Autodesk Fusion 360 part; units mm, degrees
note: some values were not read from the file. Set by a fixed rule: which face or edge a step refers to.
(part 2 of 2)
  arc A108 (60.8901, 189.5825) -> (60.8901, 183.9175) centre (63.7145, 186.75) ccw construction
  line L109 (60.8901, 189.5825) -> (63.3611, 192.0464) construction
  arc A109 (70.1855, 189.2139) -> (63.3611, 192.0464) centre (66.1855, 189.2139) ccw construction
  line L110 (70.1855, 153.7139) -> (70.1855, 148.7861) construction
  arc A110 (63.3611, 145.9536) -> (70.1855, 148.7861) centre (66.1855, 148.7861) ccw construction
  line L111 (63.3611, 145.9536) -> (60.8901, 148.4175) construction
  arc A111 (60.8901, 154.0825) -> (60.8901, 148.4175) centre (63.7145, 151.25) ccw construction
  line L112 (60.8901, 154.0825) -> (63.3611, 156.5464) construction
  arc A112 (70.1855, 153.7139) -> (63.3611, 156.5464) centre (66.1855, 153.7139) ccw construction
  line L113 (70.1855, 118.2139) -> (70.1855, 113.2861) construction
  arc A113 (63.3611, 110.4536) -> (70.1855, 113.2861) centre (66.1855, 113.2861) ccw construction
  line L114 (63.3611, 110.4536) -> (60.8901, 112.9175) construction
  arc A114 (60.8901, 118.5825) -> (60.8901, 112.9175) centre (63.7145, 115.75) ccw construction
  line L115 (60.8901, 118.5825) -> (63.3611, 121.0464) construction
  arc A115 (70.1855, 118.2139) -> (63.3611, 121.0464) centre (66.1855, 118.2139) ccw construction
  line L116 (54.844, 98) -> (49.925, 98) construction
  arc A116 (47.1006, 104.8325) -> (49.925, 98) centre (49.925, 102) ccw construction
  line L117 (47.1006, 104.8325) -> (49.5601, 107.285) construction
  arc A117 (55.2089, 107.285) -> (49.5601, 107.285) centre (52.3845, 104.4525) ccw construction
  line L118 (55.2089, 107.285) -> (57.6684, 104.8325) construction
  arc A118 (54.844, 98) -> (57.6684, 104.8325) centre (54.844, 102) ccw construction
  circle A119 centre (52.3845, 186.75) radius 3 construction
  line L119 (43.0891, 136.3325) -> (49.5601, 142.785) construction
  arc A120 (55.2089, 142.785) -> (49.5601, 142.785) centre (52.3845, 139.9525) ccw construction
  line L120 (55.2089, 142.785) -> (61.6799, 136.3325) construction
  arc A121 (61.6799, 130.6675) -> (61.6799, 136.3325) centre (58.8555, 133.5) ccw construction
  line L121 (61.6799, 130.6675) -> (55.2089, 124.215) construction
  arc A122 (49.5601, 124.215) -> (55.2089, 124.215) centre (52.3845, 127.0475) ccw construction
  line L122 (49.5601, 124.215) -> (43.0891, 130.6675) construction
  arc A123 (43.0891, 136.3325) -> (43.0891, 130.6675) centre (45.9135, 133.5) ccw construction
  line L123 (43.0891, 207.3325) -> (49.5601, 213.785) construction
  arc A124 (55.2089, 213.785) -> (49.5601, 213.785) centre (52.3845, 210.9525) ccw construction
  line L124 (55.2089, 213.785) -> (61.6799, 207.3325) construction
  arc A125 (61.6799, 201.6675) -> (61.6799, 207.3325) centre (58.8555, 204.5) ccw construction
  line L125 (61.6799, 201.6675) -> (55.2089, 195.215) construction
  arc A126 (49.5601, 195.215) -> (55.2089, 195.215) centre (52.3845, 198.0475) ccw construction
  line L126 (49.5601, 195.215) -> (43.0891, 201.6675) construction
  arc A127 (43.0891, 207.3325) -> (43.0891, 201.6675) centre (45.9135, 204.5) ccw construction
  circle A128 centre (52.3845, 115.75) radius 3 construction
  circle A129 centre (52.3845, 151.25) radius 3 construction
  circle A130 centre (52.3845, 222.25) radius 3 construction
  line L127 (61.6799, 166.1675) -> (55.2089, 159.715) construction
  arc A131 (49.5601, 159.715) -> (55.2089, 159.715) centre (52.3845, 162.5475) ccw construction
  line L128 (49.5601, 159.715) -> (43.0891, 166.1675) construction
  arc A132 (43.0891, 171.8325) -> (43.0891, 166.1675) centre (45.9135, 169) ccw construction
  line L129 (43.0891, 171.8325) -> (49.5601, 178.285) construction
  arc A133 (55.2089, 178.285) -> (49.5601, 178.285) centre (52.3845, 175.4525) ccw construction
  line L130 (55.2089, 178.285) -> (61.6799, 171.8325) construction
  arc A134 (61.6799, 166.1675) -> (61.6799, 171.8325) centre (58.8555, 169) ccw construction
  line L131 (43.8789, 112.9175) -> (41.4079, 110.4536) construction
  arc A135 (34.5835, 113.2861) -> (41.4079, 110.4536) centre (38.5835, 113.2861) ccw construction
  line L132 (34.5835, 113.2861) -> (34.5835, 118.2139) construction
  arc A136 (41.4079, 121.0464) -> (34.5835, 118.2139) centre (38.5835, 118.2139) ccw construction
  line L133 (41.4079, 121.0464) -> (43.8789, 118.5825) construction
  arc A137 (43.8789, 112.9175) -> (43.8789, 118.5825) centre (41.0545, 115.75) ccw construction
  line L134 (-52.3845, 151.25) -> (52.3845, 151.25) construction
  line L135 (0, 222.25) -> (0, 115.75) construction
  circle A138 centre (-47.5, 151.25) radius 2.25
  circle A139 centre (-37.5, 151.25) radius 2.25
  circle A140 centre (37.5, 151.25) radius 2.25
  circle A141 centre (47.5, 151.25) radius 2.25
  line L136 (-42.5, 161.25) -> (-52.5, 161.25)
  line L137 (-52.5, 161.25) -> (-52.5, 141.25)
  line L138 (-52.5, 141.25) -> (-42.5, 141.25)
  line L139 (-42.5, 141.25) -> (-42.5, 161.25)
  line L140 (-42.5, 161.25) -> (-52.5, 141.25) construction
  line L141 (-52.5, 161.25) -> (-42.5, 141.25) construction
  line L142 (-32.5, 161.25) -> (-42.5, 161.25)
  line L143 (-42.5, 161.25) -> (-42.5, 141.25)
  line L144 (-42.5, 141.25) -> (-32.5, 141.25)
  line L145 (-32.5, 141.25) -> (-32.5, 161.25)
  line L146 (-32.5, 161.25) -> (-42.5, 141.25) construction
  line L147 (-42.5, 161.25) -> (-32.5, 141.25) construction
  line L148 (42.5, 161.25) -> (32.5, 161.25)
  line L149 (32.5, 161.25) -> (32.5, 141.25)
  line L150 (32.5, 141.25) -> (42.5, 141.25)
  line L151 (42.5, 141.25) -> (42.5, 161.25)
  line L152 (42.5, 161.25) -> (32.5, 141.25) construction
  line L153 (32.5, 161.25) -> (42.5, 141.25) construction
  line L154 (52.5, 161.25) -> (42.5, 161.25)
  line L155 (42.5, 161.25) -> (42.5, 141.25)
  line L156 (42.5, 141.25) -> (52.5, 141.25)
  line L157 (52.5, 141.25) -> (52.5, 161.25)
  line L158 (52.5, 161.25) -> (42.5, 141.25) construction
  line L159 (42.5, 161.25) -> (52.5, 141.25) construction
  line L160 (-52.5, 141.25) -> (-52.5, 90)
  line L161 (-32.5, 141.25) -> (-32.5, 90)
  line L162 (-52.5, 90) -> (-32.5, 90)
  line L163 (-32.5, 90) -> (-32.5, 161.25)
  line L164 (-32.5, 161.25) -> (-52.5, 161.25)
  line L165 (-52.5, 161.25) -> (-52.5, 90)
  line L166 (32.5, 141.25) -> (32.5, 90)
  line L167 (32.5, 90) -> (52.5, 90)
  line L168 (52.5, 90) -> (52.5, 161.25)
  line L169 (52.5, 161.25) -> (32.5, 161.25)
  line L170 (32.5, 161.25) -> (32.5, 90)
  circle A142 centre (0, 151.25) radius 25
  circle A143 centre (0, 171.25) radius 1.75
  circle A144 centre (0, 131.25) radius 1.75
  point P0 (-47.5, 151.25)
  point P1 (-37.5, 151.25)
  point P2 (37.5, 151.25)
  point P3 (47.5, 151.25)
  dimension "d75" = 4.5
  dimension "d76" = 95
  dimension "d77" = 75
  dimension "d78" = 10
  dimension "d79" = 20
  dimension "d86" = 50
  dimension "d87" = 3.5
  dimension "d88" = 40
  constraint coincident A39.centre L134.start
  constraint coincident A129.centre L134.end
  constraint coincident A81.centre L135.start
  constraint coincident A91.centre L135.end
  constraint coincident L134 P0
  constraint coincident L134 P1
  constraint coincident L134 P2
  constraint coincident L134 P3
  constraint equal A138 A139
  constraint equal A138 A140
  constraint equal A138 A141
  constraint symmetric L135 A138 A141
  constraint symmetric L135 A139 A140
  constraint horizontal L136
  constraint perpendicular L136 L137
  constraint parallel L136 L138
  constraint parallel L137 L139
  constraint coincident L140 P0
  constraint coincident L141 P0
  constraint coincident P0 A138.centre
  constraint horizontal L142
  constraint perpendicular L142 L143
  constraint parallel L142 L144
  constraint parallel L143 L145
  constraint coincident L146 P1
  constraint coincident L147 P1
  constraint coincident P1 A139.centre
  constraint equal L138 L144
  constraint equal L137 L145
  constraint horizontal L148
  constraint perpendicular L148 L149
  constraint parallel L148 L150
  constraint parallel L149 L151
  constraint coincident L152 P2
  constraint coincident L153 P2
  constraint coincident P2 A140.centre
  constraint horizontal L154
  constraint perpendicular L154 L155
  constraint parallel L154 L156
  constraint parallel L155 L157
  constraint coincident L158 P3
  constraint coincident L159 P3
  constraint coincident P3 A141.centre
  constraint equal L136 L148
  constraint equal L137 L149
  constraint equal L136 L154
  constraint equal L137 L155
  constraint coincident L10 L160.end
  constraint perpendicular L10 L160
  constraint coincident L10 L161.end
  constraint perpendicular L10 L161
  constraint horizontal L162
  constraint vertical L163
  constraint horizontal L164
  constraint vertical L165
  constraint coincident L10 L166.end
  constraint perpendicular L10 L166
  constraint horizontal L167
  constraint vertical L168
  constraint horizontal L169
  constraint vertical L170
  constraint concentric A80 A142
  constraint coincident L135 A143.centre
  constraint coincident L135 A144.centre
  constraint equal A143 A144
  constraint symmetric L134 A143 A144
  measures "d75" diameter of A138
  measures "d76" distance of P0 P3
  measures "d77" distance of P1 P2
  measures "d78" distance of L137.end L138.end
  measures "d79" distance of L136.end L137.end
  measures "d86" diameter of A142
  measures "d87" diameter of A144
  measures "d88" distance of A143.centre A144.centre
extrude "Extrude9" add sketch "Sketch11" along normal blind 8 and the other way up to surface (18 mm away) contours L136 L137 L138 L139 L143 L164 L165 | L139 L142 L143 L144 L145 L163 L164 | L138 L144 L160 L161 L162 L163 L165 | L148 L149 L150 L151 L155 L169 L170 | L151 L154 L155 L156 L157 L168 L169 | L150 L156 L166 L167 L168 L170
extrude "Extrude10" cut 2 faces at (174.5, 151.25, 48.0105) (174.5, 151.3048, -48.0125) along direction (1, 0, 0) up to surface end surface through (156.5, 90, -92) normal (-1, 0, 0) offset 0
extrude "Extrude11" add sketch "Sketch11" against normal blind 16 contours L90 A89 L91 A142 | A142
equation "d26 = 150 mm - 8 mm"
equation "d28 = -150 mm + 25 mm"
equation "d35 = -8 mm - 18 mm"
equation "d48 = -150.00 mm + 8 mm"
